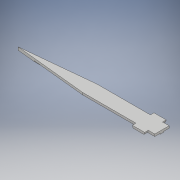
# Autodesk Inventor part: Hoja
Saved by Autodesk Inventor 2017 (Build 210142000, 142)
## iProperties
Created: 2017-01-18
Part Number: Hoja
Material: Generic
Document SubType Name: Modeling
Designer: A. Matías Quezada
Density: 1 g/cm^3
Appearance: Default
Author: A. Matías Quezada
Autodesk Inventor part; units mm, degrees
ref_plane "YZ Plane" through (0, 0, 0) normal (1, 0, 0) x (0, 1, 0)
ref_plane "XZ Plane" through (0, 0, 0) normal (0, 1, 0) x (-1, 0, 0)
ref_plane "XY Plane" through (0, 0, 0) normal (0, 0, 1) x (1, 0, 0)
sketch "Sketch1" plane through (0, 0, 0) normal (0, 0, 1) x (1, 0, 0)
  line L0 (0, 0) -> (-100, 0)
  line L1 (-100, 20) -> (0, 20)
  line L2 (0, 20) -> (0, 0)
  line L3 (-100, 20) -> (-200, 10)
  line L4 (-200, 10) -> (-100, 0)
  line L5 (-25, 25) -> (-10, 25)
  line L6 (-10, 25) -> (-10, 20)
  line L7 (-10, 20) -> (-25, 20)
  line L8 (-25, 20) -> (-25, 25)
  line L9 (-25, 0) -> (-10, 0)
  line L10 (-10, 0) -> (-10, -5)
  line L11 (-10, -5) -> (-25, -5)
  line L12 (-25, -5) -> (-25, 0)
  dimension "d0" = 100
  dimension "d1" = 20
  dimension "d2" = 200
  dimension "d3" = 10
  dimension "d4" = 15
  dimension "d5" = 5
  dimension "d6" = 10
  constraints: 26 end point, 5 parallel, 4 equal length, 3 horizontal, 3 perpendicular, 2 point on line
  measures "d0" distance of L0.start L0.end
  measures "d1" distance of L1.end L0.start
  measures "d2" horizontal distance of L1.end L3.end
  measures "d3" distance between parallel lines of L2 L10
  measures "d4" distance between parallel lines of L12 L10
  measures "d5" distance between parallel lines of L0 L11
  measures "d6" distance between parallel lines of L2 L6
extrude "Cuerpo" add sketch "Sketch1" along normal blind 3
sketch "Sketch2" plane through (0, 0, 0) normal (0, 0, -1) x (-1, 0, 0)
  line L0 (0, 0) -> (0, 20) projected
  line L1 (100, 20) -> (200, 10) projected
  line L2 (200, 10) -> (100, 0) projected
  line L3 (175, 7.5) -> (0, 7.5)
  line L4 (175, 12.5) -> (0, 12.5)
  dimension "d9" = 5
  constraints: 4 end point, 4 point on line, 2 horizontal, 1 parallel
  measures "d9" distance between parallel lines of L3 L4
extrude "Rail" add sketch "Sketch2" along normal blind 1
draft "FaceDraft1" angle -20 pull direction (0, 0, 1) faces at (-25, -1.6667, 1) fixed edges at (-25, -2.5, 0)
draft "FaceDraft2" angle -20 pull direction (0, 0, 1) faces at (-10, -3.3333, 1) fixed edges at (-10, -2.5, 0)
draft "FaceDraft3" angle -20 pull direction (0, 0, 1) faces at (-10, 21.6667, 1) fixed edges at (-10, 22.5, 0)
draft "FaceDraft4" angle -20 pull direction (0, 0, 1) faces at (-25, 23.3333, 1) fixed edges at (-25, 22.5, 0)
equation "\"d0\" = hoja_cuerpo_largo"
equation "\"d1\" = hoja_ancho"
equation "\"d2\" = hoja_largo"
equation "\"d3\" = hoja_diente_distancia"
equation "\"d4\" = hoja_diente_largo"
equation "\"d5\" = hoja_diente_ancho"
equation "\"d6\" = d3"
equation "\"d7\" = hoja_grosor"
equation "\"d9\" = hoja_rail_ancho"
equation "\"d10\" = hoja_rail_alto"
equation "\"d12\" = tirador_diente_agarre"
equation "\"d13\" = tirador_diente_agarre"
equation "\"d14\" = tirador_diente_agarre"
equation "\"d15\" = tirador_diente_agarre"
equation "\"hoja_cuerpo_largo\" = 100"
equation "\"hoja_ancho\" = 20"
equation "\"hoja_largo\" = 200"
equation "\"hoja_diente_distancia\" = 10"
equation "\"hoja_diente_largo\" = 15"
equation "\"hoja_diente_ancho\" = 5"
equation "\"hoja_grosor\" = 3"
equation "\"hoja_rail_ancho\" = 5"
equation "\"hoja_rail_alto\" = 1"
equation "\"tirador_diente_agarre\" = -20deg"
body "Solid1"
